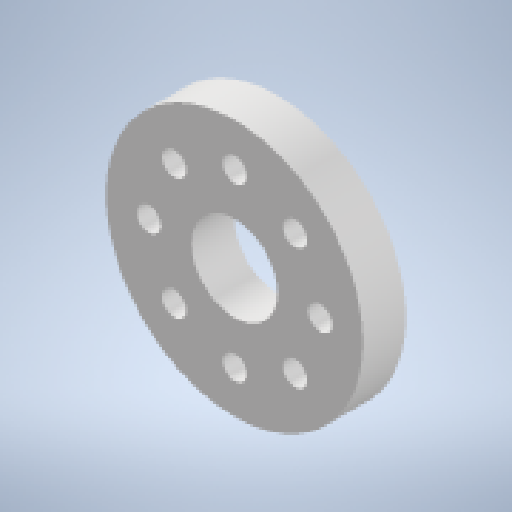
# Autodesk Inventor part: horn_3
Saved by Autodesk Inventor 2025.2 (Build 292293000, 293)
## iProperties
Created: 2025-02-13
Part Number: horn_3
Material: Generic
Document SubType Name: Modeling
Designer: Admin
Density: 1 g/cm^3
Appearance: Default
Author: Admin
Autodesk Inventor part; units mm, degrees
ref_plane "YZ Plane" through (0, 0, 0) normal (1, 0, 0) x (0, 1, 0)
ref_plane "XZ Plane" through (0, 0, 0) normal (0, 1, 0) x (-1, 0, 0)
ref_plane "XY Plane" through (0, 0, 0) normal (0, 0, 1) x (1, 0, 0)
sketch "Sketch2" plane through (0, 0, 0) normal (0, 0, 1) x (1, 0, 0)
  circle A0 centre (0, 8) radius 1.125
  circle A1 centre (0, 0) radius 1
  circle A2 centre (-5.6569, 5.6569) radius 1.125
  circle A3 centre (-8, 0) radius 1.125
  circle A4 centre (-5.6569, -5.6569) radius 1.125
  circle A5 centre (0, -8) radius 1.125
  circle A6 centre (5.6569, -5.6569) radius 1.125
  circle A7 centre (8, 0) radius 1.125
  circle A8 centre (5.6569, 5.6569) radius 1.125
  circle A9 centre (0, 0) radius 12
  circle A10 centre (0, 0) radius 4.1
  point P0 (0.1028, -10.875)
  dimension "d5" = 360
  dimension "d10" = 2.25
  dimension "d11" = 24
  dimension "d12" = 8.2
  dimension "d13" = 2
  constraints: 11 centre point, 3 coincident, 17 other
  measures "d10" diameter of A7
  measures "d11" diameter of A9
  measures "d12" diameter of A10
  measures "d13" diameter of A1
extrude "Extrusion1" add sketch "Sketch2" along normal blind 4 contours A9
sketch "Sketch5" plane through (0, 0, 4) normal (0, 0, 1) x (1, 0, 0)
  circle A0 centre (0, 0) radius 4.1
  circle A1 centre (0, 0) radius 12
  circle A2 centre (-7.9375, 0) radius 2
  circle A3 centre (-5.6127, -5.6127) radius 2
  circle A4 centre (0, -7.9375) radius 2
  circle A5 centre (5.6127, -5.6127) radius 2
  circle A6 centre (7.9375, 0) radius 2
  circle A7 centre (5.6127, 5.6127) radius 2
  circle A8 centre (0, 7.9375) radius 2
  circle A9 centre (-5.6127, 5.6127) radius 2
  dimension "d17" = 4
  dimension "d20" = 360
  constraints: 10 centre point, 2 coincident, 17 other
  measures "d17" diameter of A2
extrude "Extrusion4" add sketch "Sketch5" along normal blind 4
body "Solid1"
